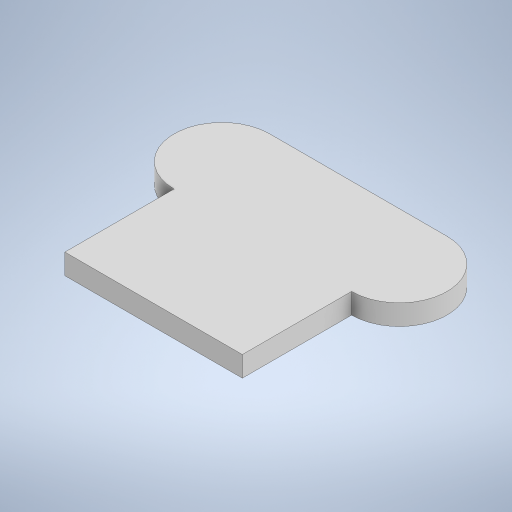
# Autodesk Inventor part: led
Saved by Autodesk Inventor 2024.1 (Build 281209000, 209)
## iProperties
Created: 2025-04-13
Part Number: led
Material: 一般
Document SubType Name: Modeling
Designer: hibik
Density: 1 g/cm^3
Appearance: 既定
Author: hibik
Autodesk Inventor part; units mm, degrees
ref_plane "YZ Plane" through (0, 0, 0) normal (1, 0, 0) x (0, 1, 0)
ref_plane "XZ Plane" through (0, 0, 0) normal (0, 1, 0) x (-1, 0, 0)
ref_plane "XY Plane" through (0, 0, 0) normal (0, 0, 1) x (1, 0, 0)
sketch "スケッチ1" plane through (0, 0, 0) normal (0, 1, 0) x (-1, 0, 0)
  line L0 (0, 0) -> (20, 0)
  line L1 (20, 0) -> (20, -15)
  line L2 (20, -15) -> (0, -15)
  line L3 (0, -15) -> (0, 0)
  circle A0 centre (16.5, -11.5) radius 3.5
  circle A1 centre (3.5, -11.5) radius 3.5
  line L4 (16.5, -11.5) -> (16.5, 0)
  line L5 (3.5, -11.5) -> (3.5, 0)
  point P0 (16.5, -15)
  point P1 (16.5, -8)
  point P2 (3.5, -8)
  point P3 (3.5, -15)
  dimension "d0" = 20
  dimension "d1" = 15
  dimension "d2" = 7
  dimension "d3" = 7
  constraints: 12 end point, 4 tangent, 3 perpendicular, 2 centre point, 2 parallel, 2 point on line, 1 horizontal
  measures "d0" distance of L1.end L2.end
  measures "d1" distance of L0.end L1.end
  measures "d2" diameter of A0
  measures "d3" diameter of A1
extrude "押し出し1" add sketch "スケッチ1" along normal blind 1.5 contours L0 L4 A0 L2 A1 L5 | A1 | A0
